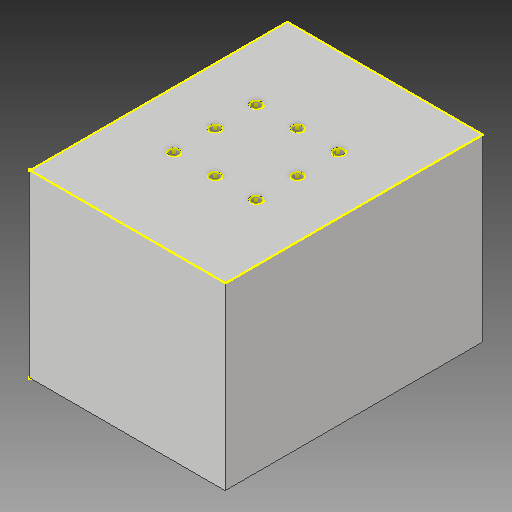
# Autodesk Inventor part: Ax12
Saved by Autodesk Inventor 2017 (Build 210142000, 142)
## iProperties
Part Number: Ax12
Material: Générique
Document SubType Name: Modeling
Designer: Thomas
Density: 1 g/cm^3
Appearance: Par défaut
Author: Thomas
Autodesk Inventor part; units mm, degrees
ref_plane "YZ Plane" through (0, 0, 0) normal (1, 0, 0) x (0, 1, 0)
ref_plane "XZ Plane" through (0, 0, 0) normal (0, 1, 0) x (-1, 0, 0)
ref_plane "XY Plane" through (0, 0, 0) normal (0, 0, 1) x (1, 0, 0)
sketch "Esquisse1" plane through (0, 0, 0) normal (1, 0, 0) x (0, 1, 0)
  line L0 (0, 0) -> (35, 0)
  line L1 (35, 0) -> (35, -50)
  line L2 (35, -50) -> (0, -50)
  line L3 (0, -50) -> (0, 0)
  dimension "d0" = 35
  dimension "d1" = 50
  constraints: 8 end point, 2 parallel, 1 horizontal, 1 perpendicular
  measures "d0" distance of L1.end L2.end
  measures "d1" distance of L0.end L1.end
extrude "Extrusion1" add sketch "Esquisse1" along normal blind 38
sketch "Esquisse2" plane through (0, 0, 0) normal (-1, 0, 0) x (0, 0, 1)
  point P0 (0, 0)
sketch "Esquisse3" plane through (0, 35, 0) normal (0, 1, 0) x (1, 0, 0)
  line L0 (0, 0) -> (38, 0) construction
  line L1 (19, 0) -> (19, 25) construction
  line L2 (0, 0) -> (0, 50) construction
  line L3 (0, 50) -> (0, 0) construction
  line L4 (0, 25) -> (11, 25) construction
  circle A0 centre (11, 25) radius 1
  line L5 (11, 25) -> (11, 17) construction
  circle A1 centre (11, 17) radius 1
  circle A2 centre (11, 25) radius 1
  circle A3 centre (11, 33) radius 1
  circle A4 centre (19, 17) radius 1
  circle A5 centre (19, 25) radius 1
  circle A6 centre (19, 33) radius 1
  circle A7 centre (27, 17) radius 1
  circle A8 centre (27, 25) radius 1
  circle A9 centre (27, 33) radius 1
  dimension "d4" = 25
  dimension "d6" = 11
  dimension "d7" = 2
  dimension "d8" = 8
  dimension "d9" = 2
  dimension "d12" = 8
  dimension "d15" = 8
  constraints: 10 centre point, 6 end point, 3 vertical, 2 coincident, 2 horizontal, 2 midpoint, 16 other
  measures "d4" distance of L1.start L1.end
  measures "d6" distance of L4.start L4.end
  measures "d7" diameter of A0
  measures "d8" distance of L5.start L5.end
  measures "d9" diameter of A1
  measures "d12" distance of A1.centre A2.centre
  measures "d15" distance of A1.centre A4.centre
extrude "Extrusion2" cut sketch "Esquisse3" against normal blind 5 contours A0 | A1 | A3 | A4 | A6 | A7 | A8 | A9
sketch "Esquisse4" plane through (0, 35, 0) normal (0, 1, 0) x (1, 0, 0)
  circle A0 centre (27, 25) radius 1 projected
  circle A1 centre (19, 33) radius 1 projected
  circle A2 centre (11, 33) radius 1 projected
  circle A3 centre (11, 25) radius 1 projected
  circle A4 centre (11, 17) radius 1 projected
  circle A5 centre (19, 17) radius 1 projected
  circle A6 centre (27, 17) radius 1 projected
  circle A7 centre (27, 33) radius 1 projected
  line L0 (0, 0) -> (0, 50) projected
  line L1 (0, 0) -> (38, 0) projected
  line L2 (38, 50) -> (38, 0) projected
  line L3 (0, 50) -> (38, 50) projected
  point P0 (0, 0)
